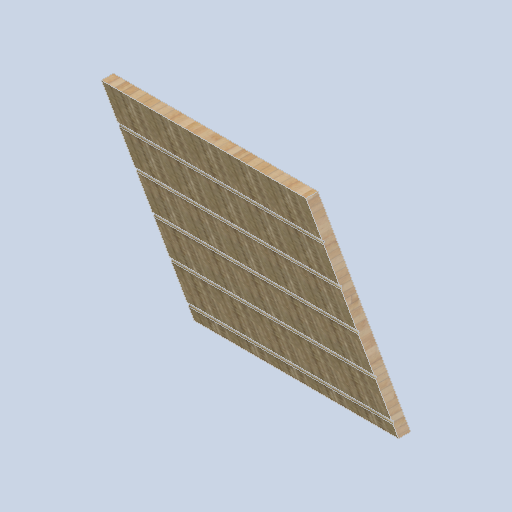
# Autodesk Inventor part: side_curve_panel_02
Saved by Autodesk Inventor 2024.2 (Build 282272000, 272)
## iProperties
Created: 2024-05-24
Part Number: side_curve_panel_02
Material: Wood (Maple)
Document SubType Name: Modeling
Designer: LOSTER_1
Density: 0.67 g/cm^3
Appearance: Natural Maple - Glossy Dark Tint
Author: LOSTER_1
Autodesk Inventor part; units mm, degrees
ref_plane "YZ Plane" through (0, 0, 0) normal (1, 0, 0) x (0, 1, 0)
ref_plane "XZ Plane" through (0, 0, 0) normal (0, 1, 0) x (-1, 0, 0)
ref_plane "XY Plane" through (0, 0, 0) normal (0, 0, 1) x (1, 0, 0)
sketch "Sketch1" plane through (0, 0, 0) normal (1, 0, 0) x (0, 1, 0)
  line L0 (-1143.0823, -35.5862) -> (966.1492, 732.1113)
  line L1 (-1143.0823, -35.5862) -> (-1143.0823, -135.5862)
  line L2 (966.1492, 732.1113) -> (966.1492, 632.1113)
  line L3 (-1143.0823, -135.5862) -> (966.1492, 632.1113)
  point P0 (0, 0)
  point P1 (1136.1492, -719.9922)
  constraints: 8 end point
extrude "Extrusion1" add sketch "Sketch1" along normal blind 1696
sketch "Sketch2" plane through (1696, 0, 0) normal (1, 0, 0) x (0, 0, -1)
  line L0 (-632.1113, 966.1492) -> (-732.1113, 966.1492) projected
  line L1 (-732.1113, 966.1492) -> (-595.3032, 590.2722)
  line L2 (-595.3032, 590.2722) -> (-585.3032, 590.2722)
  line L3 (-585.3032, 590.2722) -> (-578.4628, 571.4783)
  line L4 (-578.4628, 571.4783) -> (-588.4628, 571.4783)
  line L5 (-588.4628, 571.4783) -> (-451.6548, 195.6013)
  line L6 (-732.1113, 966.1492) -> (35.5862, -1143.0823) projected
  line L7 (-451.6548, 195.6013) -> (-441.6548, 195.6013)
  line L8 (-441.6548, 195.6013) -> (-434.8144, 176.8074)
  line L9 (-434.8144, 176.8074) -> (-445.1891, 177.8369)
  line L10 (-445.1891, 177.8369) -> (-308.381, -198.0401)
  line L11 (-308.381, -198.0401) -> (-298.381, -198.0401)
  line L12 (-298.381, -198.0401) -> (-291.5406, -216.834)
  line L13 (-291.5406, -216.834) -> (-301.5406, -216.834)
  line L14 (-301.5406, -216.834) -> (-164.7326, -592.711)
  line L15 (-164.7326, -592.711) -> (-154.7326, -592.711)
  line L16 (-154.7326, -592.711) -> (-147.8921, -611.5049)
  line L17 (-147.8921, -611.5049) -> (-157.8921, -611.5049)
  line L18 (-157.8921, -611.5049) -> (-21.0841, -987.3819)
  line L19 (-21.0841, -987.3819) -> (-11.0841, -987.3819)
  line L20 (-11.0841, -987.3819) -> (-4.2437, -1006.1758)
  line L21 (-4.2437, -1006.1758) -> (-14.2437, -1006.1758)
  line L22 (-14.2437, -1006.1758) -> (-595.3032, 590.2722)
  point P0 (0, 0)
  point P1 (-582.1113, 966.1492)
  dimension "d2" = 400
  dimension "d3" = 10
  dimension "d4" = 110
  dimension "d5" = 20
  dimension "d6" = 110
  dimension "d7" = 400
  dimension "d8" = 10
  dimension "d9" = 20
  dimension "d10" = 400
  dimension "d11" = 20
  dimension "d12" = 400
  dimension "d13" = 20
  dimension "d14" = 400
  dimension "d15" = 20
  constraints: 42 end point, 7 parallel, 4 point on line, 3 horizontal, 10 other
  measures "d2" distance of L0.end L1.end
  measures "d3" distance of L1.end L2.end
  measures "d4" angle of L2 L1
  measures "d5" distance of L2.end L3.end
  measures "d6" angle of L2 L3
  measures "d7" distance of L4.end L5.end
  measures "d8" distance of L5.end L7.end
  measures "d9" distance of L7.end L8.end
  measures "d10" distance of L9.end L10.end
  measures "d11" distance of L11.end L12.end
  measures "d12" distance of L13.end L14.end
  measures "d13" distance of L15.end L16.end
  measures "d14" distance of L17.end L18.end
  measures "d15" distance of L19.end L20.end
extrude "Extrusion2" cut sketch "Sketch2" against normal through all
fillet "Fillet1" radius 10 10 edges at (848, -1006.1758, 14.2437) (848, -987.3819, 21.0841) (848, -611.5049, 157.8921) (848, -592.711, 164.7326) (848, -216.834, 301.5406) (848, -198.0401, 308.381) (848, 177.8369, 445.1891) (848, 195.6013, 451.6548) (848, 571.4783, 588.4628) (848, 590.2722, 595.3032)
body "Solid1"
